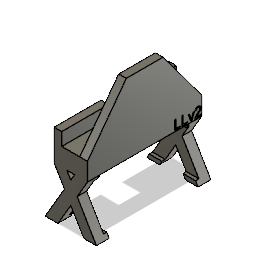
Playground Holder v2 (Autodesk Fusion 360 design; units mm, degrees)
Autodesk Fusion 360 part; units mm, degrees
sketch "Sketch1" plane through (0, 0, 0) normal (0, 1, 0) x (1, 0, 0)
  line L0 (6.5, 22.225) -> (-6.5, 22.225)
  line L1 (-6.5, 22.225) -> (-6.5, -22.225)
  line L2 (-6.5, -22.225) -> (6.5, -22.225)
  line L3 (6.5, -22.225) -> (6.5, 22.225)
  line L4 (6.5, 22.225) -> (-6.5, -22.225) construction
  line L5 (-6.5, 22.225) -> (6.5, -22.225) construction
  dimension "d1" = 44.45
  dimension "d2" = 13
extrude "Extrude1" add sketch "Sketch1" along normal blind 7
sketch "Sketch2" plane through (0, 7, 0) normal (0, 1, 0) x (-1, 0, 0)
  line L0 (-6.5, 22.225) -> (-6.5, -22.225)
  line L1 (-6.5, -22.225) -> (6.5, -22.225)
  line L2 (6.5, -22.225) -> (6.5, 22.225)
  line L3 (6.5, 22.225) -> (-6.5, 22.225)
  line L4 (6.5, -22.225) -> (3.5, -22.225)
  line L5 (3.5, -22.225) -> (3.5, 22.225)
  line L6 (3.5, 22.225) -> (6.5, 22.225)
  line L7 (6.5, 22.225) -> (6.5, -22.225)
  dimension "d5" = 44.45
  dimension "d6" = 3
extrude "Extrude2" add sketch "Sketch2" along normal blind 5 contours L1 L2 L3 L4 L5 L6 L7
sketch "Sketch3" plane through (0, 7, 0) normal (0, 1, 0) x (-1, 0, 0)
  line L0 (3.5, -22.225) -> (3.5, 22.225)
  line L1 (3.5, 22.225) -> (-6.5, 22.225)
  line L2 (-6.5, 22.225) -> (-6.5, -22.225)
  line L3 (-6.5, -22.225) -> (3.5, -22.225)
  line L4 (-6.5, -22.225) -> (-3.5, -22.225)
  line L5 (-3.5, -22.225) -> (-3.5, 22.225)
  line L6 (-3.5, 22.225) -> (-6.5, 22.225)
  line L7 (-6.5, 22.225) -> (-6.5, -22.225)
  dimension "d9" = 44.45
  dimension "d10" = 3
extrude "Extrude3" add sketch "Sketch3" along normal blind 30 contours L1 L2 L3 L4 L5 L6 L7
sketch "Sketch4" plane through (-6.5, 0, 0) normal (-1, 0, 0) x (0, 0, 1)
  line L0 (-22.225, 0) -> (22.225, 0)
  line L1 (22.225, 0) -> (22.225, 12)
  line L2 (22.225, 12) -> (-22.225, 12)
  line L3 (-22.225, 12) -> (-22.225, 0)
  line L4 (-4, 0) -> (4, 0)
  line L5 (4, 0) -> (4, 12)
  line L6 (4, 12) -> (-4, 12)
  line L7 (-4, 12) -> (-4, 0)
  line L8 (-4, 0) -> (0, 0) construction
  line L9 (0, 0) -> (4, 0) construction
  dimension "d64" = 4
  dimension "d66" = 4
  measures "d64" distance of L8.end
  measures "d66" distance of L8.end
extrude "Extrude4" cut sketch "Sketch4" against normal blind 7 contours L0 L2 L4 L5 L6 L7
sketch "Sketch5" plane through (3.5, 0, 0) normal (-1, 0, 0) x (0, 0, 1)
  line L0 (-22.225, 7) -> (22.225, 7)
  line L1 (22.225, 7) -> (22.225, 37)
  line L2 (22.225, 37) -> (-22.225, 37)
  line L3 (-22.225, 37) -> (-22.225, 7)
  line L4 (-22.225, 7) -> (0, 37)
  line L5 (0, 37) -> (22.225, 7)
  line L6 (-22.225, 7) -> (22.225, 7)
extrude "Extrude5" cut sketch "Sketch5" against normal blind 3 contours L2 L3 L4 | L1 L2 L5
sketch "Sketch6" plane through (0, 0, 0) normal (0, -1, 0) x (1, 0, 0)
  line L0 (0.5, -4) -> (-6.5, -4)
  line L1 (-6.5, -4) -> (-6.5, -22.225)
  line L2 (-6.5, -22.225) -> (6.5, -22.225)
  line L3 (6.5, -22.225) -> (6.5, 22.225)
  line L4 (6.5, 22.225) -> (-6.5, 22.225)
  line L5 (-6.5, 22.225) -> (-6.5, 4)
  line L6 (-6.5, 4) -> (0.5, 4)
  line L7 (0.5, 4) -> (0.5, -4)
  line L8 (-6.5, -22.225) -> (-1.5, -22.225)
  line L9 (-1.5, -22.225) -> (-1.5, -17.225)
  line L10 (-1.5, -17.225) -> (-6.5, -17.225)
  line L11 (-6.5, -17.225) -> (-6.5, -22.225)
  line L12 (6.5, -22.225) -> (1.5, -22.225)
  line L13 (1.5, -22.225) -> (1.5, -17.225)
  line L14 (1.5, -17.225) -> (6.5, -17.225)
  line L15 (6.5, -17.225) -> (6.5, -22.225)
  line L16 (-22, 0) -> (28, 0) construction
  line L17 (-1.5, 17.225) -> (-6.5, 17.225)
  line L18 (-1.5, 22.225) -> (-1.5, 17.225)
  line L19 (-6.5, 22.225) -> (-1.5, 22.225)
  line L20 (-6.5, 17.225) -> (-6.5, 22.225)
  line L21 (1.5, 17.225) -> (6.5, 17.225)
  line L22 (1.5, 22.225) -> (1.5, 17.225)
  line L23 (6.5, 22.225) -> (1.5, 22.225)
  line L24 (6.5, 17.225) -> (6.5, 22.225)
  dimension "d17" = 5
  dimension "d18" = 5
  dimension "d19" = 5
  dimension "d20" = 5
sketch "Sketch7" plane through (0, 0, -22.225) normal (0, 0, -1) x (-1, 0, 0)
  line L0 (-3.5, 7) -> (-6.5, 7)
  line L1 (-6.5, 7) -> (-6.5, 0)
  line L2 (-6.5, 0) -> (6.5, 0)
  line L3 (6.5, 0) -> (6.5, 12)
  line L4 (6.5, 12) -> (3.5, 12)
  line L5 (3.5, 12) -> (3.5, 7)
  line L6 (3.5, 7) -> (-3.5, 7)
  line L7 (5, 0) -> (5, -31) construction
  line L8 (-5, 0) -> (-5, -31) construction
  line L9 (-6.5, 0) -> (5, -19.6667)
  line L10 (6.5, 0) -> (-5, -19.6667)
sweep "Sweep4" add profiles "Sketch6" path "Sketch7" along L9 section 1 contours L2 L3 L12 L13 L14 L15 | L3 L4 L21 L22 L23 L24
sweep "Sweep3" add profiles "Sketch6" path "Sketch7" along L10 section 1 contours L1 L2 L8 L9 L10 L11 | L4 L5 L17 L18 L19 L20
sketch "Sketch9" plane through (0, -19.6667, 0) normal (0, -1, 0) x (1, 0, 0)
  line L0 (5, -17.225) -> (5, -22.225)
  line L1 (5, -22.225) -> (10, -22.225)
  line L2 (10, -22.225) -> (10, -17.225)
  line L3 (10, -17.225) -> (5, -17.225)
  line L4 (-6.5, -22.225) -> (10, 22.225) construction
  line L5 (10, 22.225) -> (-6.5, 22.225) construction
  line L6 (-6.5, 22.225) -> (10, -22.225) construction
sketch "Sketch10" plane through (-6.5, 0, 0) normal (-1, 0, 0) x (0, 0, 1)
  line L0 (-4, 0) -> (-4, 12)
  line L1 (-4, 12) -> (-22.225, 12)
  line L2 (-22.225, 12) -> (-22.225, 0)
  line L3 (-22.225, 0) -> (-17.225, 0)
  line L4 (-17.225, 0) -> (-4, 0)
  line L5 (18.5, -2) -> (-18.5, -2)
  line L6 (-18.5, -2) -> (-18.5, -18)
  line L7 (-18.5, -18) -> (18.5, -18)
  line L8 (18.5, -18) -> (18.5, -2)
  line L9 (18.5, -2) -> (-18.5, -18) construction
  line L10 (-18.5, -2) -> (18.5, -18) construction
  dimension "d56" = 37
  dimension "d57" = 16
extrude "Extrude6" cut sketch "Sketch10" along normal blind 15 and the other way blind 29 contours L5 L6 L7 L8
chamfer "Chamfer1" distance 12 angle 45 1 edges at (5, 37, 0)
sketch "Sketch12" plane through (6.5, 0, 0) normal (1, 0, 0) x (0, 0, -1)
  line L0 (7.1433, 27.3577) -> (-7.1433, 27.3577)
  line L1 (-7.1433, 27.3577) -> (-22.225, 7)
  line L2 (-22.225, 7) -> (-22.225, 0)
  line L3 (-22.225, 0) -> (-17.225, 0)
  line L4 (-17.225, 0) -> (17.225, 0)
  line L5 (17.225, 0) -> (22.225, 0)
  line L6 (22.225, 0) -> (22.225, 7)
  line L7 (22.225, 7) -> (7.1433, 27.3577)
  line L8 (11.6282, 0.4135) -> (21.8406, 0.4135) construction
  line L9 (21.8406, 0.4135) -> (21.8406, 5.4135) construction
  line L10 (21.8406, 5.4135) -> (11.6282, 5.4135) construction
  line L11 (11.6282, 5.4135) -> (11.6282, 0.4135) construction
  text T0 "LLv2" font "Arial" height 5 align ink ink in box 0 x 0 at (11.6382, 0.4335) x (1, 0) y (0, 1) spacing 1 height is em
extrude "Extrude8" cut sketch "Sketch12" against normal blind 2 text T0
equation "d66 = d64"
